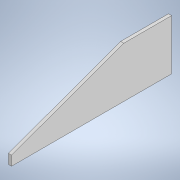
# Autodesk Inventor part: side
Saved by Autodesk Inventor 2021 (Build 250183000, 183)
## iProperties
Created: 2020-07-28
Part Number: side
Material: Generic
Document SubType Name: Modeling
Designer: johna
Density: 1 g/cm^3
Appearance: Default
Author: johna
Autodesk Inventor part; units mm, degrees
ref_plane "YZ Plane" through (0, 0, 0) normal (1, 0, 0) x (0, 1, 0)
ref_plane "XZ Plane" through (0, 0, 0) normal (0, 1, 0) x (-1, 0, 0)
ref_plane "XY Plane" through (0, 0, 0) normal (0, 0, 1) x (1, 0, 0)
sketch "Sketch1" plane through (0, 0, 0) normal (1, 0, 0) x (0, 1, 0)
  line L0 (0, 55.6574) -> (32.5774, -33.8483)
  line L1 (0, 55.6574) -> (-7.62, 55.6574)
  line L2 (-7.62, 55.6574) -> (-7.62, -33.8483)
  line L3 (32.5774, -33.8483) -> (32.5774, -71.9483)
  line L4 (32.5774, -71.9483) -> (-7.62, -71.9483)
  line L5 (-7.62, -71.9483) -> (-7.62, -33.8483)
  point P0 (0, 0)
  dimension "d1" = 95.25
  dimension "d4" = 20
  dimension "d5" = 7.62
  dimension "d6" = 38.1
  constraints: 12 end point, 2 perpendicular, 1 collinear, 1 horizontal, 1 vertical
  measures "d1" distance of L0.start L0.end
  measures "d4" angle of L2 L0
  measures "d5" distance of L0.start L1.end
  measures "d6" distance of L0.end L3.end
extrude "Extrusion1" add sketch "Sketch1" along normal blind 2.54
body "Solid1"
